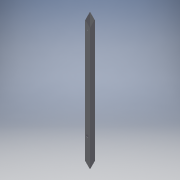
# Autodesk Inventor part: AP 3
Saved by Autodesk Inventor 2016 (Build 200138000, 138)
## iProperties
Created: 2016-02-17
Part Number: AP 3
Material: Generic
Document SubType Name: Modeling
Designer: Admin
Density: 1 g/cm^3
Appearance: Default
Author: Admin
Autodesk Inventor part; units mm, degrees
ref_plane "YZ Plane" through (0, 0, 0) normal (1, 0, 0) x (0, 1, 0)
ref_plane "XZ Plane" through (0, 0, 0) normal (0, 1, 0) x (-1, 0, 0)
ref_plane "XY Plane" through (0, 0, 0) normal (0, 0, 1) x (1, 0, 0)
sketch "Sketch1" plane through (0, 0, 0) normal (0, 1, 0) x (-1, 0, 0)
  line L0 (0, 0) -> (25.4, 0)
  line L1 (25.4, 0) -> (25.4, -25.4)
  line L2 (25.4, -25.4) -> (0, -25.4)
  line L3 (0, -25.4) -> (0, 0)
  line L4 (23.8125, -23.8125) -> (23.8125, -1.5875)
  line L5 (23.8125, -1.5875) -> (1.5875, -1.5875)
  line L6 (1.5875, -1.5875) -> (1.5875, -23.8125)
  line L7 (1.5875, -23.8125) -> (23.8125, -23.8125)
  dimension "d0" = 25.4
  dimension "d1" = 25.4
  dimension "d2" = 1.5875
  constraints: 16 end point, 4 parallel, 2 perpendicular, 1 horizontal, 3 other
  measures "d0" distance of L1.end L2.end
  measures "d1" distance of L0.end L1.end
  measures "d2" distance between parallel lines of L1 L4
extrude "Extrusion1" add sketch "Sketch1" along normal blind 698.5
sketch "Sketch2" plane through (-25.4, 0, 0) normal (0, 0, 1) x (1, 0, 0)
  circle A0 centre (12.7, 12.7) radius 6.35
  line L0 (25.4, 0) -> (0, 0) projected
  dimension "d5" = 12.7
  dimension "d6" = 12.7
  constraints: 1 centre point
  measures "d5" diameter of A0
  measures "d6" distance from line of A0.centre L0
extrude "Extrusion2" cut sketch "Sketch2" against normal blind 25.4
sketch "Sketch7" plane through (0, 0, -25.4) normal (0, 0, -1) x (-1, 0, 0)
  circle A0 centre (13.97, 151.892) radius 6.35
  line L0 (25.4, 0) -> (0, 0) projected
  line L1 (25.4, 0) -> (25.4, 698.5) projected
  dimension "d26" = 12.7
  dimension "d27" = 151.892
  dimension "d31" = 11.43
  constraints: 1 centre point
  measures "d26" diameter of A0
  measures "d27" distance from line of L0 A0.centre
  measures "d31" distance from line of A0.centre L1
extrude "Extrusion7" cut sketch "Sketch7" against normal blind 25.4
sketch "Sketch11" plane through (0, 0, -25.4) normal (0, 0, -1) x (-1, 0, 0)
  line L0 (0, 698.5) -> (25.4, 698.5) projected
  line L1 (0, 0) -> (0, 698.5) projected
  line L2 (0, 723.9) -> (0, 669.7136)
  arc A0 (0, 669.7136) -> (-29.6572, 670.9249) centre (-16.2109, 636.4744) ccw projected
  line L3 (-29.6572, 670.9249) -> (-33.1564, 670.9249) projected
  line L4 (-29.6572, 670.9249) -> (-33.1564, 670.9249)
  arc A1 (0, 669.7136) -> (-29.6572, 670.9249) centre (-16.2109, 636.4744) ccw
  arc A2 (0, 723.9) -> (-33.1564, 670.9249) centre (3.7035, 684.7184) ccw
  point P0 (25.4, 698.5)
  constraints: 4 end point, 4 point on circle, 2 centre point, 1 collinear, 1 concentric, 1 vertical, 1 other
extrude "Extrusion11" cut sketch "Sketch11" against normal blind 25.4
sketch "Sketch12" plane through (-25.4, 0, 0) normal (0, 0, 1) x (1, 0, 0)
  line L0 (25.4, 698.5) -> (0, 698.5) projected
  circle A0 centre (12.7, 673.1) radius 3.175
  circle A1 centre (12.7, 622.3) radius 3.175
  point P0 (25.4, 0)
  dimension "d46" = 6.35
  dimension "d47" = 25.4
  dimension "d48" = 6.35
  dimension "d50" = 76.2
  constraints: 2 centre point
  measures "d46" diameter of A0
  measures "d47" distance from line of L0 A0.centre
  measures "d48" diameter of A1
  measures "d50" distance from line of L0 A1.centre
extrude "Extrusion12" cut sketch "Sketch12" against normal blind 1.5875
body "Solid1"
